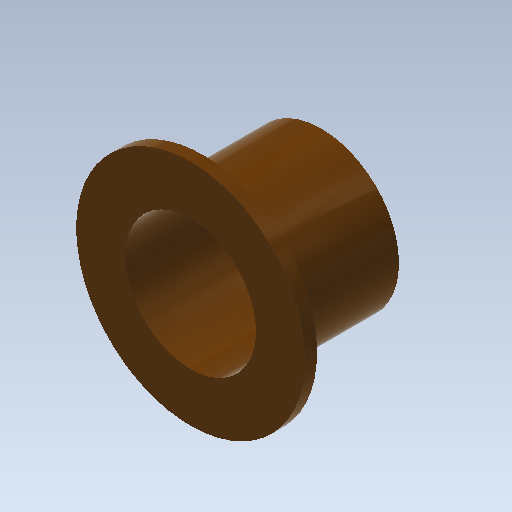
# Autodesk Inventor part: H1FI-0809-16
Saved by Autodesk Inventor 2020 (Build 240168000, 168)
## iProperties
Created: 2016-11-11
Part Number: H1FI-0809-16
Material: Generic
Document SubType Name: Modeling
Designer: jous
Density: 1 g/cm^3
Appearance: Default
Mass: 0.90442 g
Surface Area: 16.5719 cm^2
Volume: 0.90442 cm^3
Author: jous
Autodesk Inventor part; units mm, degrees
ref_plane "YZ Plane" through (0, 0, 0) normal (1, 0, 0) x (0, 1, 0)
ref_plane "XZ Plane" through (0, 0, 0) normal (0, 1, 0) x (-1, 0, 0)
ref_plane "XY Plane" through (0, 0, 0) normal (0, 0, 1) x (1, 0, 0)
sketch "Sketch1" plane through (0, 0, 0) normal (0, 0, 1) x (1, 0, 0)
  circle A0 centre (0, 0) radius 6.35
  circle A1 centre (0, 0) radius 7.5406
  dimension "d0" = 12.7
  dimension "d1" = 15.0813
  constraints: 2 centre point, 2 coincident
  measures "d0" diameter of A0
  measures "d1" diameter of A1
extrude "Extrusion1" add sketch "Sketch1" along normal blind 11.5316
sketch "Sketch2" plane through (0, 0, 11.5316) normal (0, 0, 1) x (1, 0, 0)
  circle A0 centre (0, 0) radius 6.35 projected
  circle A1 centre (0, 0) radius 7.5406 projected
  circle A2 centre (0, 0) radius 6.35
  circle A3 centre (0, 0) radius 11.1125
  dimension "d4" = 22.225
  constraints: 2 centre point, 2 coincident, 1 concentric
  measures "d4" diameter of A3
extrude "Extrusion2" add sketch "Sketch2" along normal blind 1.1684 contours A1 | A3
body "Solid1"
